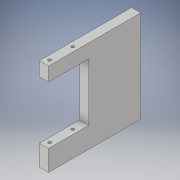
# Autodesk Inventor part: GripperPlate
Saved by Autodesk Inventor 2019 (Build 230136000, 136)
## iProperties
Created: 2019-10-02
Part Number: GripperPlate
Material: Generic
Document SubType Name: Modeling
Designer: james
Density: 1 g/cm^3
Appearance: Default
Mass: 4.85187 g
Surface Area: 34.9632 cm^2
Volume: 4.85187 cm^3
Author: james
Autodesk Inventor part; units mm, degrees
ref_plane "YZ Plane" through (0, 0, 0) normal (1, 0, 0) x (0, 1, 0)
ref_plane "XZ Plane" through (0, 0, 0) normal (0, 1, 0) x (-1, 0, 0)
ref_plane "XY Plane" through (0, 0, 0) normal (0, 0, 1) x (1, 0, 0)
sketch "Sketch1" plane through (0, 0, 0) normal (0, 1, 0) x (-1, 0, 0)
  line L0 (-1.44, 28.0571) -> (-11.6, 28.0571)
  line L1 (-11.6, 28.0571) -> (-11.6, -73.5429)
  line L2 (-11.6, -73.5429) -> (-1.44, -73.5429)
  line L3 (-1.44, -73.5429) -> (-1.44, 28.0571)
  point P0 (0, 0)
  dimension "d0" = 101.6
  dimension "d1" = 10.16
  constraints: 8 end point, 2 parallel, 1 horizontal, 1 perpendicular
  measures "d0" distance of L2.end L0.start
  measures "d1" distance between parallel lines of L1 L3
extrude "Extrusion1" add sketch "Sketch1" along normal blind 101.6
sketch "Sketch2" plane through (0, 101.6, 0) normal (0, 1, 0) x (1, 0, 0)
  line L0 (1.44, -28.0571) -> (11.6, -28.0571) projected
  point P0 (0, 0)
  point P1 (6.5886, -21.7071)
  point P2 (6.5886, 3.6929)
  dimension "d4" = 0
  dimension "d5" = 6.35
  dimension "d6" = 25.4
  measures "d4" horizontal distance of point (6.589, -21.707) point (6.589, 3.693)
  measures "d5" distance from line of L0 point (6.589, -21.707)
  measures "d6" distance of point (6.589, -21.707) point (6.589, 3.693)
hole "Hole1" at (6.5886, 101.6, 21.7071) at (6.5886, 101.6, -3.6929) direction (0, -1, 0) diameter 3.2766 end through all clearance for "Flat Head Machine Screw (82)" size "#4" standard "Ansi Unified Screw Threads"
sketch "Sketch3" plane through (11.6, 0, 28.0571) normal (1, 0, 0) x (0, 0, -1)
  line L0 (12.7, 86.36) -> (-33.0221, 86.36)
  line L1 (-33.0221, 86.36) -> (-33.0221, 22.86)
  line L2 (-33.0221, 22.86) -> (12.7, 22.86)
  line L3 (12.7, 22.86) -> (12.7, 86.36)
  line L4 (0, 101.6) -> (101.6, 101.6) projected
  line L5 (0, 0) -> (0, 101.6) projected
  point P0 (28.0571, 0)
  dimension "d15" = 15.24
  dimension "d16" = 63.5
  dimension "d19" = 12.7
  constraints: 8 end point, 2 parallel, 1 horizontal, 1 perpendicular
  measures "d15" distance between parallel lines of L4 L0
  measures "d16" distance of L0.end L1.end
  measures "d19" distance between parallel lines of L3 L5
extrude "Extrusion2" cut sketch "Sketch3" against normal blind 25.4
sketch "Sketch4" plane through (11.6, 0, 28.0571) normal (1, 0, 0) x (0, 0, -1)
  line L0 (12.7, 22.86) -> (44.45, 22.86)
  line L1 (44.45, 22.86) -> (44.45, 86.36)
  line L2 (44.45, 86.36) -> (12.7, 86.36)
  line L3 (12.7, 86.36) -> (12.7, 22.86)
  line L4 (0, 86.36) -> (12.7, 86.36) projected
  line L5 (12.7, 22.86) -> (0, 22.86) projected
  line L6 (12.7, 86.36) -> (12.7, 22.86) projected
  point P0 (28.0571, 0)
  dimension "d20" = 31.75
  dimension "d21" = 0
  dimension "d22" = 0
  dimension "d23" = 0
  constraints: 8 end point, 2 parallel, 1 horizontal, 1 perpendicular
  measures "d20" distance between parallel lines of L3 L1
  measures "d21" distance between parallel lines of L4 L2
  measures "d22" distance between parallel lines of L5 L0
  measures "d23" distance between parallel lines of L6 L3
extrude "Extrusion3" cut sketch "Sketch4" against normal blind 25.4
body "Solid1"
